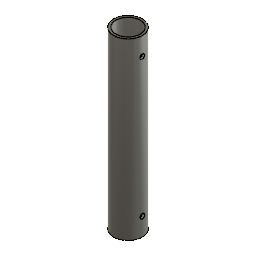
foot-assembly+(new) (Autodesk Fusion 360 archive; units mm, degrees)
design "current-leg"
Autodesk Fusion 360 part; units mm, degrees
sketch "Sketch1" plane through (0, 0, 0) normal (0, 1, 0) x (1, 0, 0)
  circle A0 centre (0, 0) radius 6.35
  dimension "d1" = 12.7
  constraint coincident A0.centre origin
  measures "d1" diameter of A0
extrude "Extrude1" add sketch "Sketch1" along normal blind 76.7
shell "Shell1" thickness 1 removed faces 1 at (0.4605, 0, -1.9232)
hole "Hole1" at (6.35, 68.7, 0) direction (-1, 0, 0) diameter 2 depth 2 tip angle 118
hole "Hole2" at (6.35, 8, 0) direction (-1, 0, 0) diameter 2 depth 2 tip angle 118
hole "Hole3" at (0, 75.7, 0) direction (0, 1, 0) diameter 10.7 depth 2 tip angle 118

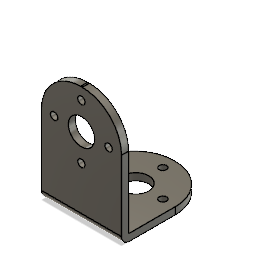
design "leg-bracket"
Autodesk Fusion 360 part; units mm, degrees
sketch "Sketch1" plane through (0, 0, 0) normal (0, 1, 0) x (1, 0, 0)
  line L0 (12, 0) -> (12.5, 0)
  line L1 (24.5, -12) -> (24.5, -28.5)
  line L2 (24.5, -28.5) -> (0, -28.5)
  line L3 (0, -28.5) -> (0, -12)
  arc A0 (12, 0) -> (0, -12) centre (12, -12) ccw
  arc A1 (24.5, -12) -> (12.5, 0) centre (12.5, -12) ccw
  point P0 (24.5, 0)
  dimension "d1" = 24.5
  dimension "d2" = 28.5
  dimension "d3" = 12
  dimension "d4" = 12
  constraint horizontal L0
  constraint vertical L1
  constraint horizontal L2
  constraint vertical L3
  constraint coincident origin L0
  constraint coincident origin L3
  constraint tangent L0 A0
  constraint tangent L3 A0
  constraint coincident P0 L0
  constraint coincident P0 L1
  constraint tangent L0 A1
  constraint tangent L1 A1
  measures "d1" distance of origin P0
  measures "d2" distance of origin L2.end
  measures "d3" radius of A0
  measures "d4" radius of A1
extrude "Extrude1" add sketch "Sketch1" along normal blind 2.2 makes body 1
hole "Hole1" at (12.25, 2.2, 11.9) direction (0, -1, 0) diameter 8 depth 13 tip angle 118 bodies 1
hole "Hole2" at (12.25, 2.2, 3.575) direction (0, -1, 0) diameter 2.25 depth 13 tip angle 118 bodies 1
hole "Hole3" at (20.575, 2.2, 11.9) direction (0, -1, 0) diameter 2.25 depth 13 tip angle 118 bodies 1
hole "Hole4" at (3.925, 2.2, 11.9) direction (0, -1, 0) diameter 2.25 depth 13 tip angle 118 bodies 1
hole "Hole5" at (12.25, 2.2, 20.225) direction (0, -1, 0) diameter 2.25 depth 13 tip angle 118 bodies 1
copy_body "CopyPasteBodies1" bodies 1 makes body 2
move_body "Move1" bodies 2 to x (1, 0, 0) y (0, 0, 1) z (0, -1, 0) at (0, 28.5, 26.3)
move_body "Move3" bodies 2 to x (1, 0, 0) y (0, 1, 0) z (0, 0, 1) at (0, 7.55, 0)
extrude "Extrude2" add 1 faces at (16.3333, 7.55, 27.7667) along direction (0, -1, 0) blind 6 on bodies 2 bodies 2 1
fillet "Fillet1" radius 2.5 1 edges at (12.25, 0, 28.5) on bodies 2

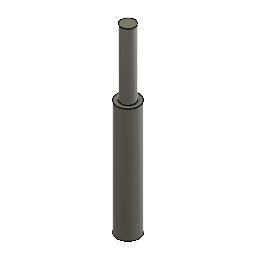
design "Camera"
Autodesk Fusion 360 part; units mm, degrees
sketch "Sketch1" plane through (0, 0, 0) normal (0, 1, 0) x (1, 0, 0)
  circle A0 centre (5, -5) radius 3.675
  dimension "d1" = 7.35
  measures "d1" diameter of A0
extrude "Extrude1" add sketch "Sketch1" along normal blind 38.1
sketch "Sketch2" plane through (0, 38.1, 0) normal (0, 1, 0) x (-1, 0, 0)
  circle A0 centre (-5, 5) radius 3.675
  circle A1 centre (-5, 5) radius 2.3
  dimension "d4" = 4.6
  constraint concentric A0 A1
  measures "d4" diameter of A1
extrude "Extrude2" add sketch "Sketch2" along normal blind 22 contours A1
sketch "Sketch3" plane through (0, 0, 0) normal (0, 1, 0) x (1, 0, 0)
  circle A0 centre (5, -5) radius 1.75
  dimension "d7" = 3.5
  measures "d7" diameter of A0
extrude "Extrude3" cut sketch "Sketch3" along normal blind 1

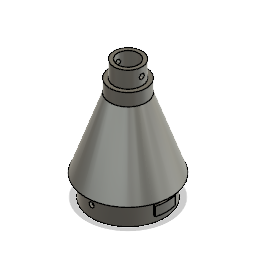
design "Foot-cone"
Autodesk Fusion 360 part; units mm, degrees
sketch "Sketch1" plane through (0, 0, 0) normal (0, 0, 1) x (1, 0, 0)
  line L0 (0, 0) -> (0, 30)
  line L1 (0, 0) -> (-12.3, 0)
  line L2 (0, 30) -> (-3.75, 30)
  line L3 (-5.1, 30) -> (-5.1, 36)
  line L4 (-15.5, 0) -> (-13.3, 0)
  line L5 (-3.75, 30) -> (-3.75, 36)
  line L6 (-3.75, 36) -> (-5.1, 36)
  line L7 (-5.1, 30) -> (-6.6, 30)
  line L8 (-12.3, 0) -> (-3.88, 29)
  line L9 (-15.5, 0) -> (-6.6, 25.4545)
  line L10 (-6.6, 30) -> (-6.6, 25.4545)
  line L11 (-13.3, 0) -> (-13.3, -7.7)
  line L12 (-13.3, -7.7) -> (-12.3, -7.7)
  line L13 (-12.3, -7.7) -> (-12.3, 0)
  line L14 (-3.75, 30) -> (-2.6, 30)
  line L15 (-2.6, 30) -> (-2.6, 29)
  line L16 (-2.6, 29) -> (-3.88, 29)
  line L17 (-13.3, -1.9995) -> (-14.1, -1.9995)
  line L18 (-14.1, -1.9995) -> (-14.1, -5.2995)
  line L19 (-14.1, -5.2995) -> (-13.3, -5.2995)
  dimension "d1" = 30
  dimension "d2" = 13.3
  dimension "d3" = 3.75
  dimension "d5" = 1.5
  dimension "d14" = 0.8
  dimension "d15" = 3.3
  constraint coincident L0.start L1.start
  constraint vertical L0
  constraint perpendicular L0 L1
  constraint perpendicular L0 L2
  constraint perpendicular L1 L3
  constraint parallel L1 L4
  constraint perpendicular L2 L5
  constraint perpendicular L3 L6
  constraint perpendicular L3 L7
  constraint perpendicular L7 L10
  constraint perpendicular L4 L11
  constraint perpendicular L11 L12
  constraint perpendicular L1 L13
  constraint coincident L2 L14.end
  constraint perpendicular L2 L15
  constraint perpendicular L15 L16
  constraint coincident L11 L17.start
  constraint perpendicular L11 L17
  constraint perpendicular L17 L18
  constraint coincident L11 L19.end
  constraint perpendicular L11 L19
  measures "d1" distance of L0.start L0.end
  measures "d2" distance of L0.start L4.end
  measures "d3" distance of L0.end L2.end
  measures "d5" distance of L3.start L7.end
  measures "d14" distance of L17.start L17.end
  measures "d15" distance of L17.end L18.end
revolve "Revolve1" add sketch "Sketch1" angle 360 about axis through (0, 0, 0) along (0, 1, 0) contours L2 L3 L4 L5 L6 L7 L8 L9 L10 L11 L12 L13 L14 L15 L16 makes body 1
hole "Hole1" at (5.1, 33, 0) direction (-1, 0, 0) diameter 1.8 depth 5 tip angle 118 bodies 1
hole "Hole2" at (-5.1, 33, 0) direction (1, 0, 0) diameter 1.8 depth 5 tip angle 118 bodies 1
revolve "Revolve2" add sketch "Sketch1" angle 30 about axis through (0, 30, 0) along (0, 1, 0) contours L11 L17 L18 L19 bodies 1
revolve "Revolve3" add sketch "Sketch1" angle 30 about axis through (0, 30, 0) along (0, -1, 0) separate body contours L11 L17 L18 L19 makes body 2
move_body "Move1" bodies 2 to x (-0.866025, 0, 0.5) y (0, 1, 0) z (-0.5, 0, -0.866025) at (0, 0, 0)
combine "Combine1" operation add target body 1 tool bodies 2
move_face "MoveFace1" to x (0.965926, 0, 0.258819) y (0, 1, 0) z (-0.258819, 0, 0.965926) at (0, 0, 0) 10 faces at (-12.2519, -1.9995, 6.3653) (-14.0866, -4.1995, 0.615) (-13.5667, -4.1995, 0) (-11.7491, -4.1995, 6.7833) (-12.2519, -5.2995, 6.3653) (13.595, -5.2995, -2.4086) (11.7491, -4.1995, -6.7833) (13.595, -1.9995, -2.4086) (12.5069, -4.1995, -6.5107) (13.5667, -4.1995, 0) on bodies 1
hole "Hole3" at (0, -3.5, 13.3) direction (0, 0, -1) diameter 1.8 depth 5 tip angle 118 bodies 1

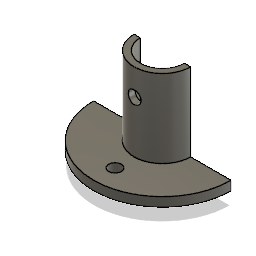
design "joint-split-leg"
Autodesk Fusion 360 part; units mm, degrees
sketch "Sketch1" plane through (0, 0, 0) normal (0, 1, 0) x (1, 0, 0)
  circle A0 centre (0, 0) radius 11.9
  dimension "d1" = 23.8
  constraint coincident A0.centre origin
  measures "d1" diameter of A0
extrude "Extrude1" add sketch "Sketch1" along normal blind 1.6 makes body 1
sketch "Sketch2" plane through (0, 1.6, 0) normal (0, 1, 0) x (-1, 0, 0)
  circle A0 centre (0, 0) radius 11.9
  circle A1 centre (0, 0) radius 4.9
  dimension "d4" = 9.8
  constraint coincident A0.centre A1.centre
  measures "d4" diameter of A1
extrude "Extrude2" add sketch "Sketch2" along normal blind 13.5 contours A1 bodies 1
sketch "Sketch3" plane through (0, 15.1, 0) normal (0, 1, 0) x (-1, 0, 0)
  circle A0 centre (0, 0) radius 4.9
  circle A1 centre (0, 0) radius 2.3
  dimension "d7" = 4.6
  constraint concentric A0 A1
  measures "d7" diameter of A1
extrude "Extrude3" cut sketch "Sketch3" against normal blind 20 contours A1 bodies 1
sketch "Sketch4" plane through (0, 0, 0) normal (0, -1, 0) x (1, 0, 0)
  circle A0 centre (0, 0) radius 2.3
  circle A1 centre (0, 0) radius 11.9
  circle A2 centre (0, 0) radius 3.925
  dimension "d10" = 7.85
  constraint coincident A0.centre A1.centre
  measures "d10" diameter of A2
extrude "Extrude4" add sketch "Sketch4" along normal blind 2.2 contours A2 bodies 1
sketch "Sketch6" plane through (0, 1.6, 0) normal (0, 1, 0) x (-1, 0, 0)
  circle A0 centre (0, 0) radius 4.9
  circle A1 centre (0, 0) radius 11.9
  circle A2 centre (0, -8.2) radius 1.1
  dimension "d16" = 2.2
  measures "d16" diameter of A2
hole "Hole2" at (0, 1.6, -8.2) direction (0, -1, 0) diameter 2.2 depth 1.6 tip angle 118 bodies 1
move_face "MoveFace1" to x (-1, 0, 0) y (0, 1, 0) z (0, 0, -1) at (0, 0, 0) 1 faces at (0.0548, 1.0667, -7.1014) on bodies 1
hole "Hole3" at (0, 1.6, -8.2) direction (0, -1, 0) diameter 2.2 depth 1.6 tip angle 118 bodies 1
hole "Hole4" at (0, 9.685, 4.9) direction (0, 0, -1) diameter 2.2 depth 11 tip angle 118 bodies 1
move_face "MoveFace2" to x (1, 0, 0) y (0, 1, 0) z (0, 0, 1) at (0, 0.855, 0) 2 faces at (0.0576, 10.7835, 4.0325) (0.0519, 10.7837, -4.0326) on bodies 1
sketch "Sketch7" plane through (0, 1.6, 0) normal (0, 1, 0) x (-1, 0, 0)
  circle A0 centre (0, 0) radius 3.8
  dimension "d30" = 7.6
  constraint coincident A0.centre origin
  measures "d30" diameter of A0
extrude "Extrude5" cut sketch "Sketch7" along normal blind 13.5 bodies 1
sketch "Sketch8" plane through (0, 1.6, 0) normal (0, 1, 0) x (-1, 0, 0)
  circle A0 centre (0, -8.2) radius 1.1
  circle A1 centre (0, 8.2) radius 1.1
  circle A2 centre (0, 0) radius 4.9
  circle A3 centre (0, 0) radius 11.9
  line L0 (11.9, 0) -> (-11.9, 0)
  constraint coincident A3 L0.start
  constraint coincident A3 L0.end
  constraint horizontal L0
fillet "Fillet1" radius 0.85 1 edges at (-2.1444, -2.2, 0.8317) on bodies 1
split "Split1" by curves path "Sketch8" along L0 bodies 1 makes body 2 at (-3.6302, 0, 6.7235)
hidden bodies 1
